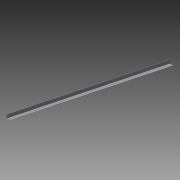
# Autodesk Inventor part: Front Right Beam
Saved by Autodesk Inventor 2015 (Build 190159000, 159)
## iProperties
Created: 2015-01-10
Part Number: Front Right Beam
Material: Generic
Document SubType Name: Modeling
Designer: Chandler Willoughby
Density: 1 g/cm^3
Appearance: Default
Author: Chandler Willoughby
Autodesk Inventor part; units mm, degrees
ref_plane "YZ Plane" through (0, 0, 0) normal (1, 0, 0) x (0, 1, 0)
ref_plane "XZ Plane" through (0, 0, 0) normal (0, 1, 0) x (-1, 0, 0)
ref_plane "XY Plane" through (0, 0, 0) normal (0, 0, 1) x (1, 0, 0)
sketch "Sketch1" plane through (0, 0, 0) normal (0, 1, 0) x (-1, 0, 0)
  line L0 (0, 0) -> (1893.3131, 0) construction
  line L1 (0, 0) -> (1149.4728, 0) construction
  line L2 (-482.6, -1828.8) -> (0, 0)
  line L3 (0, 0) -> (-50.8, 0)
  line L4 (-482.6, -1828.8) -> (-533.4, -1828.8)
  line L5 (-533.4, -1828.8) -> (-50.8, 0)
  constraints: 12 end point, 4 horizontal
extrude "Extrusion1" add sketch "Sketch1" along normal blind 3.175
sketch "Sketch2" plane through (0, 3.175, 0) normal (0, 1, 0) x (1, 0, 0)
  line L0 (0, 0) -> (3.175, 0)
  line L1 (0, 0) -> (50.8, 0) projected
  line L2 (0, 0) -> (482.6, 1828.8)
  line L3 (482.6, 1828.8) -> (0, 0) projected
  line L4 (482.6, 1828.8) -> (485.775, 1828.8)
  line L5 (533.4, 1828.8) -> (482.6, 1828.8) projected
  line L6 (485.775, 1828.8) -> (3.175, 0)
  dimension "d9" = 3.175
  dimension "d10" = 3.175
  constraints: 8 end point, 2 point on line, 1 collinear
  measures "d9" distance of L0.start L0.end
  measures "d10" distance of L2.end L4.end
extrude "Extrusion2" add sketch "Sketch2" along normal blind 47.625
body "Solid1"
